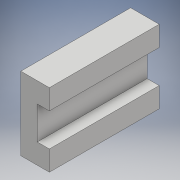
# Autodesk Inventor part: linear_SSEB10
Saved by Autodesk Inventor 2018.3 (Build 223284000, 284)
## iProperties
Created: 2018-05-22
Part Number: linear_SSEB10
Material: 一般
Document SubType Name: Modeling
Designer: Shin
Density: 1 g/cm^3
Appearance: 既定
Author: Shin
Autodesk Inventor part; units mm, degrees
ref_plane "YZ Plane" through (0, 0, 0) normal (1, 0, 0) x (0, 1, 0)
ref_plane "XZ Plane" through (0, 0, 0) normal (0, 1, 0) x (-1, 0, 0)
ref_plane "XY Plane" through (0, 0, 0) normal (0, 0, 1) x (1, 0, 0)
sketch "スケッチ1" plane through (0, 0, 0) normal (0, 1, 0) x (-1, 0, 0)
  line L0 (0, 0) -> (7.8, 0)
  line L1 (7.8, 0) -> (7.8, -20)
  line L2 (7.8, -20) -> (0, -20)
  line L3 (0, -20) -> (0, 0)
  line L4 (0, -5.5) -> (3.3, -5.5)
  line L5 (3.3, -5.5) -> (3.3, -14.5)
  line L6 (3.3, -14.5) -> (0, -14.5)
  line L7 (0, -14.5) -> (0, -5.5)
  dimension "d0" = 7.8
  dimension "d1" = 20
  dimension "d2" = 3.3
  dimension "d3" = 9
  dimension "d4" = 5.5
  constraints: 16 end point, 4 parallel, 2 horizontal, 2 perpendicular, 1 point on line
  measures "d0" distance of L1.end L2.end
  measures "d1" distance of L0.end L1.end
  measures "d2" distance of L5.end L6.end
  measures "d3" distance of L4.end L5.end
  measures "d4" distance between parallel lines of L0 L4
extrude "押し出し1" add sketch "スケッチ1" along normal blind 30 contours L0 L1 L2 L3 L6 L5 L4
sketch "スケッチ2" plane through (-7.8, 0, -20) normal (-1, 0, 0) x (0, 0, 1)
  line L0 (17.5, 30.0313) -> (17.5, 0)
  line L1 (2.5, 30.0313) -> (2.5, 0)
  line L2 (20, 0) -> (20, 30) projected
  line L3 (0, 0) -> (0, 30) projected
  line L4 (0, 30) -> (20, 30) projected
  point P0 (2.5, 20)
  point P1 (2.5, 10)
  point P2 (17.5, 20)
  point P3 (17.5, 10)
  dimension "d7" = 2.5
  dimension "d8" = 2.5
  dimension "d9" = 10
  dimension "d10" = 10
  dimension "d11" = 10
  dimension "d12" = 10
  constraints: 4 end point, 4 point on line, 2 vertical
  measures "d7" distance between parallel lines of L2 L0
  measures "d8" distance between parallel lines of L3 L1
  measures "d9" distance from line of L4 point (17.5, 20)
  measures "d10" distance of point (17.5, 10) point (17.5, 20)
  measures "d11" distance of point (2.5, 20) point (2.5, 10)
  measures "d12" distance from line of L4 point (2.5, 20)
hole "穴1" at (-7.8, 20, -17.5) at (-7.8, 10, -17.5) at (-7.8, 20, -2.5) at (-7.8, 10, -2.5) direction (1, 0, 0) diameter 3 depth 3 tip angle 118
